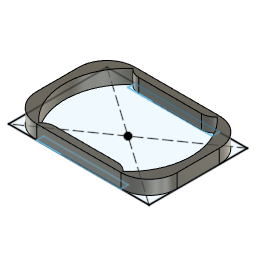
KeyChain (Autodesk Fusion 360 design; units mm, degrees)
Autodesk Fusion 360 part; units mm, degrees
note: some values were not read from the file. Chosen so that the rebuilt part matches the saved one: which bodies a step acts on.
sketch "Keychain Sketch" plane through (0, 0, 0) normal (0, 0, 1) x (1, 0, 0)
  line L0 (50, 35) -> (-50, 35)
  line L1 (-50, 35) -> (-50, -35)
  line L2 (-50, -35) -> (50, -35)
  line L3 (50, -35) -> (50, 35)
  line L4 (50, 35) -> (-50, -35) construction
  line L5 (-50, 35) -> (50, -35) construction
  dimension "d1" = 70
  dimension "d2" = 100
  constraint perpendicular L0 L1
  constraint parallel L0 L2
  constraint parallel L1 L3
  constraint horizontal L0
  constraint coincident L4 origin
  constraint coincident L5 origin
  measures "d1" distance of L0.end L1.end
  measures "d2" distance of L1.end L2.end
extrude "Extrude1" add sketch "Keychain Sketch" along normal blind 10 makes body 1
hole "Hole1" at (0, 0, 10) direction (0, 0, -1) diameter 90 depth 40 tip angle 118 bodies 1 makes body 2 at (29.9816, -33.5574, 3.3333)
sketch "KeychainSide" plane through (0, 0, 0) normal (0, 0, 1) x (1, 0, 0)
  line L0 (-30, 35) -> (30, 35)
  line L1 (-30, 35) -> (-30, 30)
  line L2 (-30, 30) -> (30, 30)
  line L3 (30, 30) -> (30, 35)
  line L4 (-30, -30) -> (30, -30)
  line L5 (-30, -30) -> (-30, -35)
  line L6 (-30, -35) -> (30, -35)
  line L7 (30, -35) -> (30, -30)
  constraint horizontal L0
  constraint perpendicular L0 L1
  constraint perpendicular L1 L2
  constraint perpendicular L0 L3
  constraint horizontal L4
  constraint perpendicular L4 L5
  constraint perpendicular L5 L6
  constraint perpendicular L4 L7
extrude "Extrude3" add sketch "KeychainSide" along normal blind 10 contours L4 L5 L6 L7 bodies 1 2
extrude "Extrude2" add sketch "KeychainSide" along normal blind 10 contours L0 L1 L2 L3 bodies 1
fillet "Fillet1" radius 10 1 edges at (-30, 30, 5) on bodies 1
fillet "Fillet2" radius 10 1 edges at (30, 30, 5) on bodies 1
fillet "Fillet3" radius 10 1 edges at (30, -30, 5) on bodies 1
fillet "Fillet4" radius 10 1 edges at (-30, -30, 5) on bodies 1
fillet "Fillet5" radius 20 1 edges at (50, -35, 5) on bodies 1
fillet "Fillet6" radius 20 3 edges at (50, 35, 5) (-50, -35, 5) (-50, 35, 5) on bodies 1
named bodies: "KeyChain"
